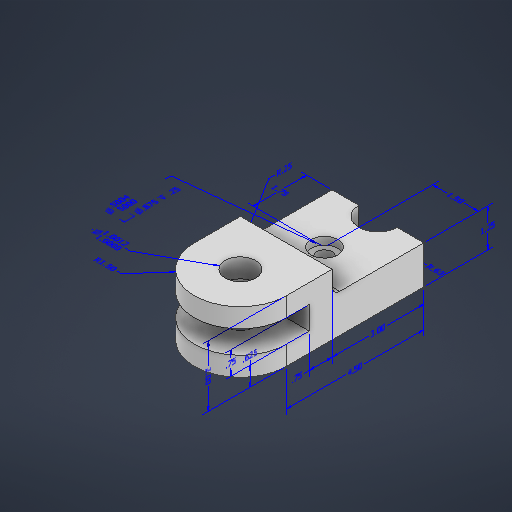
# Autodesk Inventor part: pivot_lock
Saved by Autodesk Inventor 2026.2 (Build 302298010, 298A)
## iProperties
Created: 2025-03-10
Part Number: pivot_lock
Material: Generic
Document SubType Name: Modeling
Designer: a00584475
Density: 1 g/cm^3
Appearance: Default
Author: a00584475
Autodesk Inventor part; units mm, degrees
ref_plane "YZ Plane" through (0, 0, 0) normal (1, 0, 0) x (0, 1, 0)
ref_plane "XZ Plane" through (0, 0, 0) normal (0, 1, 0) x (-1, 0, 0)
ref_plane "XY Plane" through (0, 0, 0) normal (0, 0, 1) x (1, 0, 0)
sketch "Sketch1" plane through (0, 0, 0) normal (0, 1, 0) x (-1, 0, 0)
  line L0 (0, 0) -> (0, -114.3)
  line L1 (0, -114.3) -> (76.2, -114.3)
  line L2 (76.2, -114.3) -> (76.2, 0)
  line L3 (76.2, 0) -> (0, 0)
  dimension "d0" = 114.3
  dimension "d1" = 76.2
  constraints: 8 end point, 3 perpendicular, 1 vertical
  measures "d0" distance of L0.start L0.end
  measures "d1" distance of L0.end L1.end
extrude "REC 1" add sketch "Sketch1" along normal blind 31.75
sketch "Sketch2" plane through (0, 31.75, 0) normal (0, 1, 0) x (1, 0, 0)
  line L0 (-76.2, 0) -> (0, 0) projected
  line L1 (0, 0) -> (0, 38.1)
  line L2 (0, 0) -> (0, 114.3) projected
  line L3 (0, 38.1) -> (-76.2, 38.1)
  line L4 (-76.2, 114.3) -> (-76.2, 0) projected
  line L5 (-76.2, 38.1) -> (-76.2, 0)
  line L6 (-76.2, 0) -> (0, 0)
  dimension "d4" = 38.1
  constraints: 8 end point, 2 perpendicular, 1 horizontal, 1 point on line
  measures "d4" distance of L0.end L1.end
extrude "REC 2" add sketch "Sketch2" along normal blind 19.05
fillet "Face Fillet1" radius 6.35 1 edges at (-38.1, 31.75, -38.1)
sketch "Sketch3" plane through (0, 31.75, 0) normal (0, 1, 0) x (1, 0, 0)
  line L0 (0, 114.3) -> (-76.2, 114.3) projected
  circle A0 centre (-38.1, 114.3) radius 15.875
  point P0 (0, 0)
  dimension "d8" = 15.875
  constraints: 1 centre point, 1 midpoint
  measures "d8" radius of A0
extrude "C CUT -  RIGHT" cut sketch "Sketch3" against normal through all
sketch "Sketch5" plane through (0, 50.8, 0) normal (0, 1, 0) x (1, 0, 0)
  line L0 (-76.2, 0) -> (0, 0) projected
  arc A0 (-76.2, 0) -> (0, 0) centre (-38.1, 0) ccw
  line L1 (0, 0) -> (-76.2, 0)
  constraints: 2 end point, 2 point on circle, 1 centre point, 1 collinear, 1 midpoint
extrude "Extrusion5" cut sketch "Sketch5" against normal blind 19.05
sketch "Sketch6" plane through (0, 50.8, 0) normal (0, 1, 0) x (1, 0, 0)
  line L0 (-76.2, 0) -> (0, 0) projected
  arc A0 (-76.2, 0) -> (0, 0) centre (-38.1, 0) ccw
  constraints: 2 point on circle, 1 centre point, 1 midpoint
extrude "TOP ARC" add sketch "Sketch6" against normal blind 15.875
sketch "Sketch7" plane through (0, 0, 0) normal (0, -1, 0) x (1, 0, 0)
  line L0 (0, 0) -> (-76.2, 0) projected
  arc A0 (0, 0) -> (-76.2, 0) centre (-38.1, 0) ccw
  constraints: 2 point on circle, 1 centre point, 1 midpoint
extrude "BOTTOM ARC" add sketch "Sketch7" against normal blind 15.875
sketch "Sketch8" plane through (0, 50.8, 0) normal (0, 1, 0) x (1, 0, 0)
  circle A0 centre (-38.1, 0) radius 12.7
  line L0 (0, 0) -> (-76.2, 0) projected
  line L1 (0, 38.1) -> (-76.2, 38.1) projected
  line L2 (-76.2, 38.1) -> (-76.2, 0) projected
  point P0 (-38.1, 38.1)
  dimension "d21" = 25.4
  dimension "d25" = 38.1
  dimension "d26" = 38.1
  constraints: 2 midpoint, 1 centre point
  measures "d21" diameter of A0
  measures "d25" distance of point (-38.1, 38.1) A0.centre
  measures "d26" distance from line of L2 A0.centre
extrude "HOLE - LEFT" cut sketch "Sketch8" against normal through all
sketch "Sketch4" plane through (0, 31.75, 0) normal (0, 1, 0) x (1, 0, 0)
  circle A0 centre (-38.1, 69.85) radius 6.35
  line L0 (-53.975, 114.3) -> (-76.2, 114.3) projected
  point P0 (0, 0)
  dimension "d11" = 44.45
  dimension "d12" = 12.7
  constraints: 1 centre point
  measures "d11" distance from line of L0 A0.centre
  measures "d12" diameter of A0
extrude "HOLE - RIGHT" cut sketch "Sketch4" against normal through all
sketch "Sketch9" plane through (0, 31.75, 0) normal (0, 1, 0) x (1, 0, 0)
  circle A0 centre (-38.1, 69.85) radius 6.35 projected
  circle A1 centre (-38.1, 69.85) radius 11.1125
  point P0 (0, 0)
  dimension "d27" = 22.225
  constraints: 1 centre point, 1 coincident
  measures "d27" diameter of A1
extrude "BIGGER HOLE - RIGHT" cut sketch "Sketch9" against normal blind 6.35
sketch "Sketch10" plane through (0, 0, -114.3) normal (1, 0, 0) x (0, 0, -1)
  line L0 (-114.3, 15.875) -> (-114.3, 34.925) projected
  line L1 (-114.3, 34.925) -> (-95.25, 34.925)
  line L2 (-95.25, 34.925) -> (-95.25, 15.875)
  line L3 (-95.25, 15.875) -> (-114.3, 15.875)
  line L4 (-114.3, 15.875) -> (-114.3, 34.925)
  point P0 (-114.3, 0)
  dimension "d44" = 19.05
  constraints: 8 end point, 2 parallel, 1 horizontal, 1 perpendicular
  measures "d44" distance of L2.end L3.end
extrude "Extrusion10" cut sketch "Sketch10" against normal through all
body "Solid1"
